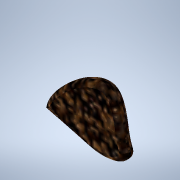
# Autodesk Inventor part: Obstacle stone
Saved by Autodesk Inventor 2021 (Build 250183000, 183)
## iProperties
Created: 2021-07-08
Part Number: Obstacle stone
Material: Generic
Document SubType Name: Modeling
Designer: shifa
Density: 1 g/cm^3
Appearance: Default
Author: shifa
Autodesk Inventor part; units mm, degrees
ref_plane "YZ Plane" through (0, 0, 0) normal (1, 0, 0) x (0, 1, 0)
ref_plane "XZ Plane" through (0, 0, 0) normal (0, 1, 0) x (-1, 0, 0)
ref_plane "XY Plane" through (0, 0, 0) normal (0, 0, 1) x (1, 0, 0)
sketch "Sketch1" plane through (0, 0, 0) normal (0, 0, 1) x (1, 0, 0)
  line L0 (0, 0) -> (2.7316, 18.4533) construction
  line L1 (2.7316, 18.4533) -> (38.9049, 39.4847) construction
  line L2 (38.9049, 39.4847) -> (38.9049, 0) construction
  line L3 (38.9049, 0) -> (35.2981, 0) construction
  line L4 (35.2981, 0) -> (35.2981, -6.2852) construction
  line L5 (35.2981, -6.2852) -> (20.4026, -6.2852) construction
  line L6 (20.4026, -6.2852) -> (18.6034, -4.5921) construction
  line L7 (18.6034, -4.5921) -> (0, 0) construction
  spline S0 degree 4 poles (0, 0) (2.7316, 18.4533) (38.9049, 39.4847) (38.9049, 0) (35.2981, 0) (35.2981, -6.2852) (20.4026, -6.2852) (18.6034, -4.5921) (0, 0) knots 1 1 1 1 1 2 3 4 5 6 6 6 6 6
  constraints: 2 horizontal, 2 vertical, 2 other
extrude "Extrusion1" add sketch "Sketch1" along normal blind 5
fillet "Fillet2" radius 2 2 edges at (35.9697, -1.1232, 5) (35.9697, -1.1232, 0)
body "Solid1"
